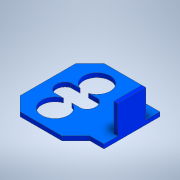
# Autodesk Inventor part: Ultrasonic_Body
Saved by Autodesk Inventor 2021 (Build 250183000, 183)
## iProperties
Created: 2024-06-09
Part Number: Ultrasonic_Body
Material: Generic
Document SubType Name: Modeling
Designer: User
Density: 1 g/cm^3
Appearance: Default
Author: User
Autodesk Inventor part; units mm, degrees
ref_plane "YZ Plane" through (0, 0, 0) normal (1, 0, 0) x (0, 1, 0)
ref_plane "XZ Plane" through (0, 0, 0) normal (0, 1, 0) x (-1, 0, 0)
ref_plane "XY Plane" through (0, 0, 0) normal (0, 0, 1) x (1, 0, 0)
sketch "Sketch1" plane through (0, 0, 0) normal (0, 1, 0) x (-1, 0, 0)
  line L0 (0, 0) -> (30, 0)
  line L1 (0, 0) -> (-30, 0)
  line L2 (30, 0) -> (-10, 0)
  line L3 (-10, 0) -> (-10, 30)
  line L4 (-10, 0) -> (-10, -30)
  line L5 (-10, 30) -> (20, 30)
  line L6 (-10, -30) -> (20, -30)
  line L7 (20, 30) -> (20, -30)
  line L8 (30, 0) -> (30, 20)
  line L9 (30, 0) -> (30, -20)
  line L10 (30, 20) -> (20, 30)
  line L11 (30, -20) -> (20, -30)
  line L12 (-30, 0) -> (-30, 20)
  line L13 (-30, 0) -> (-30, -20)
  line L14 (-30, 20) -> (-20, 20)
  line L15 (-20, 20) -> (-10, 30)
  line L16 (-30, -20) -> (-20, -20)
  line L17 (-20, -20) -> (-10, -30)
  line L18 (20, 0) -> (20, 6)
  line L19 (20, 0) -> (20, -6)
  arc A0 (20, -6) -> (20, 6) centre (17.6853, 0) ccw
  line L20 (0, 0) -> (0, 6)
  line L21 (0, 0) -> (0, -6)
  arc A1 (0, 6) -> (0, -6) centre (2.3147, 0) ccw
  line L22 (0, 30) -> (10, 30)
  circle A2 centre (10.0225, 15.038) radius 9
  line L23 (0, -30) -> (10, -30)
  circle A3 centre (10, -15) radius 9
  line L24 (20, 6) -> (20, -6)
  line L25 (20, 6) -> (0, 6)
  line L26 (20, -6) -> (0, -6)
  point P0 (10, -6)
  dimension "d0" = 30
  dimension "d1" = 30
  dimension "d2" = 40
  dimension "d5" = 30
  dimension "d6" = 30
  dimension "d8" = 30
  dimension "d9" = 30
  dimension "d10" = 20
  dimension "d11" = 20
  dimension "d12" = 20
  dimension "d13" = 20
  dimension "d14" = 10
  dimension "d15" = 10
  dimension "d16" = 6
  dimension "d17" = 6
  dimension "d18" = 6.431
  dimension "d19" = 6
  dimension "d20" = 6
  dimension "d22" = 6.431
  dimension "d25" = 18
  dimension "d28" = 18
  constraints: 54 end point, 7 point on line, 6 horizontal, 6 vertical, 4 centre point, 4 point on circle, 2 perpendicular, 1 collinear, 1 midpoint
  measures "d0" distance of L0.start L0.end
  measures "d1" distance of L0.start L1.end
  measures "d2" distance of L0.end L2.end
  measures "d5" distance of L2.end L3.end
  measures "d6" distance of L2.end L4.end
  measures "d8" distance of L3.end L5.end
  measures "d9" distance of L4.end L6.end
  measures "d10" distance of L0.end L8.end
  measures "d11" distance of L0.end L9.end
  measures "d12" distance of L1.end L12.end
  measures "d13" distance of L1.end L13.end
  measures "d14" distance of L12.end L14.end
  measures "d15" distance of L13.end L16.end
  measures "d16" distance of L18.start L18.end
  measures "d17" distance of L18.start L19.end
  measures "d18" radius of A0
  measures "d19" distance of L0.start L20.end
  measures "d20" distance of L0.start L21.end
  measures "d22" radius of A1
  measures "d25" diameter of A2
  measures "d28" diameter of A3
extrude "Extrusion1" add sketch "Sketch1" along normal blind 3 contours A1 L26 L7 L6 L4 L1 | L1 L3 L5 L7 L25 A1 | A0 L7 L10 L8 L0 | L0 L9 L11 L7 A0 | L4 L17 L16 L13 L1 | L1 L12 L14 L15 L3
sketch "Sketch2" plane through (0, 3, 0) normal (0, 1, 0) x (1, 0, 0)
  line L0 (30, 10) -> (30, -10)
  line L1 (30, 10) -> (27, 10)
  line L2 (27, 10) -> (27, -10)
  line L3 (27, -10) -> (30, -10)
  line L4 (-19, -30) -> (-10, -30)
  circle A0 centre (-10, -15) radius 9.5
  circle A1 centre (-10, 15) radius 9.5
  point P0 (0, 0)
  dimension "d34" = 20
  dimension "d35" = 3
  dimension "d37" = 19
  dimension "d39" = 19
  constraints: 10 end point, 2 centre point, 2 perpendicular, 1 horizontal
  measures "d34" distance of L0.start L0.end
  measures "d35" distance of L0.start L1.end
  measures "d37" diameter of A0
  measures "d39" diameter of A1
hole "Hole1" at (-10, 3, 15) direction (0, -1, 0) diameter 19 end through all
hole "Hole2" at (-10, 3, -15) direction (0, -1, 0) diameter 19 end through all
sketch "Sketch3" plane through (0, 3, 0) normal (0, 1, 0) x (1, 0, 0)
  line L0 (30, 10) -> (30, -10)
  line L1 (30, -10) -> (27, -10)
  line L2 (27, -10) -> (27, 10)
  line L3 (27, 10) -> (30, 10)
  point P0 (0, 0)
  constraints: 8 end point, 3 perpendicular
extrude "Extrusion2" add sketch "Sketch3" along normal blind 20
body "Solid1"
